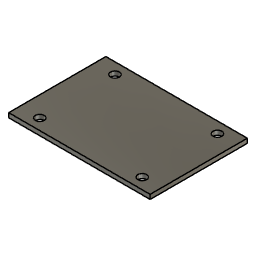
Raspberry Pi Debug Probe v0 (Autodesk Fusion 360 design; units mm, degrees)
Autodesk Fusion 360 part; units mm, degrees
sketch "Sketch1" plane through (0, 0, 0) normal (0, 0, 1) x (1, 0, 0)
  line L0 (0, 0) -> (32.01, 0)
  line L1 (32.01, 0) -> (32.01, 22)
  line L2 (32.01, 22) -> (0, 22)
  line L3 (0, 22) -> (0, 0)
  dimension "d1" = 32.01
  dimension "d2" = 22
  constraint horizontal L0
  constraint vertical L1
  constraint horizontal L2
  constraint vertical L3
  constraint coincident L0.start L3.end
  measures "d1" distance of L0.start L0.end
  measures "d2" distance of L0.start L2.end
extrude "Extrude1" add sketch "Sketch1" along normal blind 1
sketch "Sketch3" plane through (0, 0, 1) normal (0, 0, 1) x (-1, 0, 0)
  line L0 (0, -22) -> (0, 0)
  line L1 (0, 0) -> (-32.01, 0)
  line L2 (-32.01, 0) -> (-32.01, -22)
  line L3 (-32.01, -22) -> (0, -22)
  circle A0 centre (-4.55, -19.5) radius 1
  circle A1 centre (-27.75, -19.5) radius 1
  circle A2 centre (-4.55, -2.49) radius 1
  circle A3 centre (-27.75, -2.49) radius 1
  dimension "d5" = 2
  dimension "d6" = 2.5
  dimension "d7" = 4.55
  dimension "d10" = -23.2
  dimension "d11" = 17.01
  measures "d5" diameter of A0
  measures "d6" distance of L3 A0.centre
  measures "d7" distance of L0 A0.centre
extrude "Extrude2" cut sketch "Sketch3" against normal blind 1 contours A0 | A1 | A2 | A3
